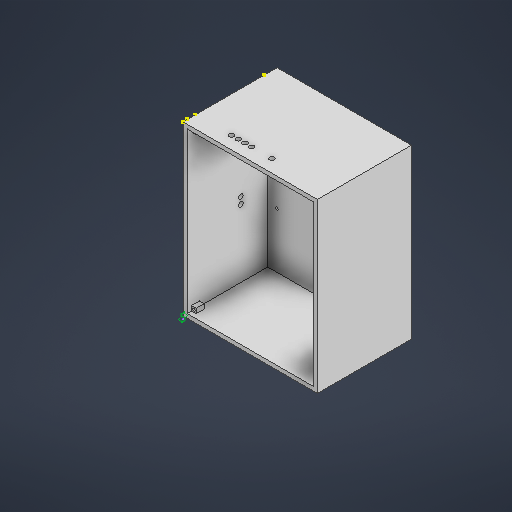
# Autodesk Inventor part: base
Saved by Autodesk Inventor 2026.3 (Build 303398000, 398)
## iProperties
Created: 2026-05-13
Part Number: base
Material: Genérico
Document SubType Name: Modeling
Designer: Santiago A
Density: 1 g/cm^3
Appearance: Valor por defecto
Author: Santiago A
Autodesk Inventor part; units mm, degrees
ref_plane "YZ Plane" through (0, 0, 0) normal (1, 0, 0) x (0, 1, 0)
ref_plane "XZ Plane" through (0, 0, 0) normal (0, 1, 0) x (-1, 0, 0)
sketch "Boceto3" plane through (0, 0, 0) normal (0, 0, 1) x (1, 0, 0)
  line L0 (0, 0) -> (100, 0)
  line L1 (100, 0) -> (100, -125)
  line L2 (100, -125) -> (0, -125)
  line L3 (0, -125) -> (0, 0)
  dimension "d8" = 100
  dimension "d9" = 125
  constraints: 8 end point, 2 parallel, 1 horizontal, 1 perpendicular
  measures "d8" distance of L1.end L2.end
  measures "d9" distance of L0.end L1.end
extrude "Extrusión2" add sketch "Boceto3" along normal blind 70
sketch "Boceto4" plane through (0, 0, 70) normal (0, 0, 1) x (1, 0, 0)
  line L0 (0, 0) -> (50, 0)
  line L1 (100, 0) -> (0, 0) projected
  line L2 (0, 0) -> (0, -125) projected
  line L3 (0, 0) -> (0, -45)
  line L4 (6.25, -5.5) -> (93.75, -5.5)
  line L5 (93.75, -5.5) -> (93.75, -84.5)
  line L6 (93.75, -84.5) -> (6.25, -84.5)
  line L7 (6.25, -84.5) -> (6.25, -5.5)
  line L8 (6.25, -5.5) -> (93.75, -84.5) construction
  line L9 (93.75, -5.5) -> (6.25, -84.5) construction
  line L10 (6.25, -5.5) -> (9.75, -5.5)
  line L11 (6.25, -5.5) -> (6.25, -9)
  circle A0 centre (9.75, -9) radius 1
  line L12 (93.75, -5.5) -> (90.25, -5.5)
  line L13 (93.75, -5.5) -> (93.75, -9)
  circle A1 centre (90.25, -9) radius 1
  line L14 (93.75, -84.5) -> (90.25, -84.5)
  line L15 (93.75, -84.5) -> (93.75, -81)
  circle A2 centre (90.25, -81) radius 1
  line L16 (6.25, -84.5) -> (9.75, -84.5)
  line L17 (6.25, -84.5) -> (6.25, -81)
  circle A3 centre (9.75, -81) radius 1
  point P0 (50, -45)
  dimension "d12" = 45
  dimension "d13" = 87.5
  dimension "d14" = 79
  dimension "d22" = 3.5
  dimension "d23" = 3.5
  dimension "d24" = 2
  dimension "d25" = 3.5
  dimension "d26" = 3.5
  dimension "d27" = 2
  dimension "d28" = 3.5
  dimension "d29" = 3.5
  dimension "d30" = 2
  dimension "d31" = 3.5
  dimension "d32" = 3.5
  dimension "d33" = 2
  constraints: 32 end point, 9 point on line, 4 centre point, 3 midpoint, 2 parallel, 1 horizontal, 1 perpendicular
  measures "d12" distance of L0.start L3.end
  measures "d13" distance of L5.end L6.end
  measures "d14" distance of L4.end L5.end
  measures "d22" distance of L4.start L10.end
  measures "d23" distance of L4.start L11.end
  measures "d24" diameter of A0
  measures "d25" distance of L4.end L12.end
  measures "d26" distance of L4.end L13.end
  measures "d27" diameter of A1
  measures "d28" distance of L5.end L14.end
  measures "d29" distance of L5.end L15.end
  measures "d30" diameter of A2
  measures "d31" distance of L6.end L16.end
  measures "d32" distance of L6.end L17.end
  measures "d33" diameter of A3
sketch "Boceto5" plane through (0, 0, 70) normal (0, 0, 1) x (1, 0, 0)
  line L0 (100, 0) -> (0, 0) projected
  line L1 (0, 0) -> (0, -62.5)
  line L2 (0, 0) -> (0, -125) projected
  line L3 (0, 0) -> (3, 0)
  line L4 (0, 0) -> (0, -3)
  line L5 (100, -125) -> (100, 0) projected
  line L6 (100, -125) -> (100, -122)
  line L7 (0, -125) -> (100, -125) projected
  line L8 (100, -125) -> (97, -125)
  line L9 (97, -122) -> (3, -122)
  line L10 (3, -122) -> (3, -3)
  line L11 (3, -3) -> (97, -3)
  line L12 (97, -3) -> (97, -122)
  dimension "d15" = 62.5
  dimension "d16" = 3
  dimension "d17" = 3
  dimension "d18" = 3
  dimension "d19" = 3
  constraints: 18 end point, 4 point on line, 2 parallel, 1 horizontal, 1 midpoint, 1 perpendicular
  measures "d15" distance of L0.end L1.end
  measures "d16" distance of L0.end L3.end
  measures "d17" distance of L0.end L4.end
  measures "d18" distance of L5.start L6.end
  measures "d19" distance of L5.start L8.end
extrude "Extrusión3" cut sketch "Boceto5" against normal blind 60 contours L9 L10 L11 L12
extrude "Extrusión4" cut sketch "Boceto4" against normal blind 65 contours A0 | A1 | A2 | A3
sketch "Boceto7" plane through (0, 0, 70) normal (0, 0, 1) x (1, 0, 0)
  point P0 (0, 0)
sketch "Boceto8" plane through (0, 0, 70) normal (0, 0, 1) x (1, 0, 0)
  point P0 (0, 0)
ref_plane "Plano de trabajo1" through (0, 0, 60.75) normal (0, 0, 1) x (1, 0, 0)
sketch "Boceto9" plane through (0, 0, 60.75) normal (0, 0, 1) x (1, 0, 0)
  line L0 (3, -3) -> (6.5, -3)
  line L1 (6.5, -3) -> (6.5, -6.5)
  line L2 (6.5, -6.5) -> (3, -6.5)
  line L3 (3, -6.5) -> (3, -3)
  line L4 (97.0016, -3) -> (93.5016, -3)
  line L5 (93.5016, -3) -> (93.5016, -6.5)
  line L6 (93.5016, -6.5) -> (97.0016, -6.5)
  line L7 (97.0016, -6.5) -> (97.0016, -3)
  line L8 (3, -122) -> (3, -3) projected
  line L9 (3, -122) -> (6.5, -122)
  line L10 (6.5, -122) -> (6.5, -118.5)
  line L11 (6.5, -118.5) -> (3, -118.5)
  line L12 (3, -118.5) -> (3, -122)
  line L13 (97, -3) -> (97, -122) projected
  line L14 (97, -122) -> (93.5, -122)
  line L15 (93.5, -122) -> (93.5, -118.5)
  line L16 (93.5, -118.5) -> (97, -118.5)
  line L17 (97, -118.5) -> (97, -122)
  point P0 (0, 0)
  point P1 (97, -6.5)
  dimension "d61" = 3.5
  dimension "d62" = 3.5
  dimension "d63" = 3.5
  dimension "d64" = 3.5
  dimension "d65" = 3.5
  dimension "d66" = 3.5
  dimension "d70" = 3.5
  dimension "d71" = 3.5
  constraints: 32 end point, 8 parallel, 4 horizontal, 4 perpendicular, 1 point on line
  measures "d61" distance of L1.end L2.end
  measures "d62" distance of L0.end L1.end
  measures "d63" distance of L6.end L5.end
  measures "d64" distance of L5.end L4.end
  measures "d65" distance of L11.end L10.end
  measures "d66" distance of L10.end L9.end
  measures "d70" distance of L15.end L16.end
  measures "d71" distance of L14.end L15.end
ref_plane "Plano de trabajo2" through (0, 0, 60.25) normal (0, 0, 1) x (1, 0, 0)
sketch "Boceto10" plane through (3, -122, 70) normal (0, 1, 0) x (1, 0, 0)
  point P0 (-3, 70)
sketch "Boceto11" plane through (0, 0, 10) normal (0, 0, 1) x (1, 0, 0)
  line L0 (-58.2651, -184.2292) -> (-60.7624, -188.5609)
  point P0 (0, 0)
  dimension "d68" = 5
  constraints: 2 end point
  measures "d68" distance of L0.start L0.end
sketch "Boceto12" plane through (0, 0, 60.75) normal (0, 0, 1) x (1, 0, 0)
  point P0 (0, 0)
extrude "Extrusión6" add sketch "Boceto9" along normal blind 6
sketch "Boceto13" plane through (0, 0, 66.75) normal (0, 0, 1) x (1, 0, 0)
  point P0 (0, 0)
sketch "Boceto14" plane through (0, 0, 66.75) normal (0, 0, 1) x (1, 0, 0)
  line L0 (6.5, -122) -> (6.5, -118.5) projected
  line L1 (6.5, -118.5) -> (4.75, -118.5)
  line L2 (6.5, -118.5) -> (3, -118.5) projected
  line L3 (6.5, -118.5) -> (6.5, -120.25)
  circle A0 centre (4.75, -120.25) radius 1
  line L4 (93.5, -118.5) -> (93.5, -122) projected
  line L5 (93.5, -118.5) -> (95.25, -118.5)
  line L6 (97, -118.5) -> (93.5, -118.5) projected
  line L7 (93.5, -118.5) -> (93.5, -120.25)
  circle A1 centre (95.25, -120.25) radius 1
  line L8 (3, -3) -> (97, -3) projected
  line L9 (97, -3) -> (95.25, -3)
  line L10 (97, -3) -> (97, -4.75)
  line L11 (97, -3) -> (97, -122) projected
  circle A2 centre (95.25, -4.75) radius 1
  line L12 (3, -122) -> (3, -3) projected
  line L13 (3, -3) -> (4.75, -3)
  line L14 (3, -3) -> (3, -4.75)
  circle A3 centre (4.75, -4.75) radius 1
  point P0 (0, 0)
  dimension "d74" = 1.75
  dimension "d75" = 1.75
  dimension "d76" = 2
  dimension "d77" = 1.75
  dimension "d78" = 1.75
  dimension "d79" = 2
  dimension "d80" = 1.75
  dimension "d81" = 1.75
  dimension "d82" = 2
  dimension "d83" = 1.75
  dimension "d84" = 1.75
  dimension "d85" = 2
  constraints: 16 end point, 4 centre point, 4 midpoint, 4 point on line
  measures "d74" distance of L0.end L1.end
  measures "d75" distance of L0.end L3.end
  measures "d76" diameter of A0
  measures "d77" distance of L4.start L5.end
  measures "d78" distance of L4.start L7.end
  measures "d79" diameter of A1
  measures "d80" distance of L8.end L9.end
  measures "d81" distance of L8.end L10.end
  measures "d82" diameter of A2
  measures "d83" distance of L8.start L13.end
  measures "d84" distance of L8.start L14.end
  measures "d85" diameter of A3
extrude "Extrusión7" cut sketch "Boceto14" against normal blind 4
sketch "Boceto15" plane through (0, 0, 66.75) normal (0, 0, 1) x (1, 0, 0)
  point P0 (0, 0)
sketch "Boceto16" plane through (3, -122, 70) normal (1, 0, 0) x (0, 0, -1)
  line L0 (60, 0) -> (60, 119) projected
  line L1 (60, 50.4292) -> (40, 50.4292)
  line L2 (60, 50.4292) -> (80, 50.4292) construction
  circle A0 centre (40, 50.4292) radius 1.75
  line L3 (40, 50.4292) -> (40, 55.4292)
  circle A1 centre (40, 55.4292) radius 1.75
  point P0 (70, 122)
  dimension "d88" = 20
  dimension "d89" = 180
  dimension "d90" = 3.5
  dimension "d91" = 5
  dimension "d92" = 3.5
  constraints: 6 end point, 2 centre point, 2 coincident, 1 collinear, 1 horizontal, 1 perpendicular, 1 point on line, 1 vertical
  measures "d88" distance of L1.start L1.end
  measures "d89" angle of L1 L2
  measures "d90" diameter of A0
  measures "d91" distance of L3.start L3.end
  measures "d92" diameter of A1
extrude "Extrusión8" cut sketch "Boceto16" against normal blind 10
sketch "Boceto17" plane through (3, -3, 70) normal (0, -1, 0) x (1, 0, 0)
  line L0 (0, -60) -> (94, -60) projected
  line L1 (23.6532, -59.4188) -> (73.6532, -59.4188) construction
  circle A0 centre (23.6532, -9.4188) radius 1.75
  circle A1 centre (28.6532, -9.4188) radius 1.75
  circle A2 centre (33.6532, -9.4188) radius 1.75
  circle A3 centre (38.6532, -9.4188) radius 1.75
  circle A4 centre (53.6532, -9.4188) radius 1.75
  point P0 (-3, -70)
  dimension "d97" = 3.5
  dimension "d99" = 3.5
  dimension "d101" = 3.5
  dimension "d103" = 3.5
  dimension "d109" = 3.5
  constraints: 5 centre point, 2 end point, 1 horizontal
  measures "d97" diameter of A0
  measures "d99" diameter of A1
  measures "d101" diameter of A2
  measures "d103" diameter of A3
  measures "d109" diameter of A4
extrude "Extrusión9" cut sketch "Boceto17" against normal blind 10
